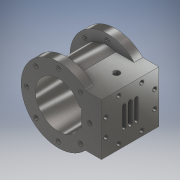
# Autodesk Inventor part: reverse gear cylinder
Saved by Autodesk Inventor 2017 (Build 210142000, 142)
## iProperties
Created: 2018-11-10
Part Number: reverse gear cylinder
Material: Generic
Document SubType Name: Modeling
Designer: User
Density: 1 g/cm^3
Appearance: Default
Author: User
Autodesk Inventor part; units mm, degrees
ref_plane "YZ Plane" through (0, 0, 0) normal (1, 0, 0) x (0, 1, 0)
sketch "Sketch2" plane through (0, 0, 0) normal (0, 1, 0) x (-1, 0, 0)
  arc A0 (-18.7617, -18) -> (-18.7617, 18) centre (0, 0) ccw
  arc A1 (-14.8324, -6) -> (-14.8324, 6) centre (0, 0) ccw
  line L0 (-16, 0) -> (-16, -6)
  line L1 (-16, 0) -> (-16, 6)
  line L2 (-16, 6) -> (-14.8324, 6) construction
  line L3 (-16, -6) -> (-14.8324, -6)
  circle A2 centre (22, 0) radius 1.5
  circle A3 centre (15.5563, 15.5563) radius 1.5
  circle A4 centre (0, 22) radius 1.5
  circle A5 centre (-15.5563, 15.5563) radius 1.5
  circle A6 centre (-22, 0) radius 1.5
  circle A7 centre (-15.5563, -15.5563) radius 1.5
  circle A8 centre (0, -22) radius 1.5
  circle A9 centre (15.5563, -15.5563) radius 1.5
  line L4 (-14.8324, 6) -> (-16, 6)
  line L5 (-30, 0) -> (-30, -18)
  line L6 (-30, -18) -> (-30, 18)
  line L7 (-30, 18) -> (-18.7617, 18)
  line L8 (-30, -18) -> (-18.7617, -18)
  arc A10 (-21.9489, 1.4991) -> (-22, 0) centre (0, 0) ccw
  line L9 (0, 0) -> (-16, 0)
  line L10 (-20.5, 0) -> (-22, 0)
  dimension "d10" = 360
  dimension "d2" = 52
  dimension "d3" = 32
  dimension "d4" = 6
  dimension "d5" = 6
  dimension "d6" = 3
  dimension "d7" = 30
  dimension "d8" = 18
  dimension "d9" = 36
  dimension "d36" = 22
  dimension "d37" = 0
  dimension "d38" = 18
  dimension "d39" = 0
  dimension "d40" = 16
  dimension "d41" = 38
  constraints: 22 end point, 11 centre point, 8 point on circle, 3 coincident, 3 equal length, 3 vertical, 2 horizontal, 2 perpendicular, 2 point on line, 2 tangent, 17 other
  measures "d2" diameter of A0
  measures "d3" diameter of A1
  measures "d4" distance of L0.start L0.end
  measures "d5" distance of L0.start L1.end
  measures "d6" diameter of A2
  measures "d7" distance of L9.start L5.start
  measures "d8" distance of L5.start L5.end
  measures "d9" distance of L5.end L6.end
  measures "d36" radius of A10
  measures "d37" distance between parallel lines of L10 L9
  measures "d38" distance between parallel lines of L9 L7
  measures "d39" distance from line of point (0, 0) L9
  measures "d40" distance from line of point (0, 0) L1
  measures "d41" distance from line of A2.centre L1
extrude "Extrusion1" add sketch "Sketch2" along normal blind 40
ref_plane "Work Plane1" through (0, 0, 0) normal (0, 1, 0) x (-1, 0, 0)
sketch "Sketch6" plane through (0, 0, 0) normal (0, 1, 0) x (-1, 0, 0)
  arc A0 (-6.0828, -18) -> (-6.0828, 18) centre (0, 0) ccw
  circle A1 centre (0, 0) radius 26
  arc A2 (-18.7617, -18) -> (-18.7617, 18) centre (0, 0) ccw
  line L0 (-18.7617, 18) -> (-6.0828, 18)
  line L1 (-18.7617, -18) -> (-6.0828, -18)
  dimension "d31" = 38
  dimension "d32" = 52
  dimension "d73" = 26
  dimension "d74" = 36
  dimension "d75" = 18
  dimension "d76" = 18
  dimension "d77" = 0
  constraints: 4 end point, 4 point on circle, 3 centre point, 2 coincident, 1 concentric, 1 horizontal, 1 parallel
  measures "d31" diameter of A0
  measures "d32" diameter of A1
  measures "d73" radius of A2
  measures "d74" distance between parallel lines of L1 L0
  measures "d75" distance from line of point (0, 0) L0
  measures "d76" distance from line of point (0, 0) L0
  measures "d77" distance of point (0, 0) A0.centre
sketch "Sketch4" plane through (30, 0, 18) normal (1, 0, 0) x (0, 0, -1)
  circle A0 centre (12, 3) radius 1.5
  circle A1 centre (3.5, 12) radius 1.5
  line L0 (0, 3) -> (0, 37) construction
  line L1 (0, 20) -> (36, 20) construction
  circle A2 centre (3.5, 28) radius 1.5
  circle A3 centre (12, 37) radius 1.5
  line L2 (16.5, 40) -> (19.5, 40) construction
  line L3 (18, 40) -> (18, 0) construction
  line L4 (19.5, 0) -> (16.5, 0) construction
  circle A4 centre (24, 37) radius 1.5
  circle A5 centre (32.5, 28) radius 1.5
  circle A6 centre (32.5, 12) radius 1.5
  circle A7 centre (24, 3) radius 1.5
  line L5 (-1, 37) -> (-1, 3)
  line L6 (37, 37) -> (37, 3)
  arc A8 (11.25, 21.5) -> (11.25, 18.5) centre (11.25, 20) ccw
  arc A9 (24.75, 18.5) -> (24.75, 21.5) centre (24.75, 20) ccw
  line L7 (24.75, 21.5) -> (24.75, 23)
  arc A10 (24.75, 23) -> (24.75, 25.5) centre (24.75, 24.25) ccw
  arc A11 (11.25, 25.5) -> (11.25, 23) centre (11.25, 24.25) ccw
  line L8 (24.75, 14.5) -> (11.25, 14.5)
  line L9 (24.75, 17) -> (11.25, 17)
  arc A12 (11.25, 17) -> (11.25, 14.5) centre (11.25, 15.75) ccw
  arc A13 (24.75, 14.5) -> (24.75, 17) centre (24.75, 15.75) ccw
  line L10 (11.25, 21.5) -> (24.75, 21.5)
  line L11 (24.75, 18.5) -> (11.25, 18.5)
  line L12 (11.25, 25.5) -> (24.75, 25.5)
  line L13 (11.25, 23) -> (24.75, 23)
  point P0 (18, 0)
  point P1 (0, 40)
  point P2 (36, 3)
  point P3 (18, 0)
  dimension "d18" = 3
  dimension "d21" = 3
  dimension "d22" = 3
  dimension "d23" = 1.5
  dimension "d24" = 2.5
  dimension "d25" = 2.5
  dimension "d26" = 2.5
  dimension "d42" = 12.25
  dimension "d43" = 19
  dimension "d44" = 37
  dimension "d45" = 38
  dimension "d46" = 25.5
  dimension "d47" = 20
  dimension "d48" = 17
  dimension "d49" = 40
  dimension "d50" = 19
  dimension "d51" = 0
  dimension "d52" = 37
  dimension "d53" = 3
  dimension "d54" = 1
  dimension "d55" = 1
  dimension "d56" = 3
  dimension "d57" = 4.5
  dimension "d58" = 28
  dimension "d59" = 12.25
  dimension "d60" = 13
  dimension "d61" = 37
  dimension "d62" = 17.5
  dimension "d63" = 17.5
  dimension "d64" = 19
  dimension "d65" = 0
  dimension "d66" = 25.75
  dimension "d67" = 25.75
  dimension "d68" = 37
  dimension "d69" = 40
  dimension "d70" = 37
  dimension "d71" = 37
  dimension "d72" = 3
  constraints: 28 end point, 14 centre point, 12 point on circle, 12 tangent, 9 parallel, 6 symmetric about line, 3 midpoint, 2 equal radius, 2 horizontal, 1 vertical, 6 other
  measures "d18" diameter of A0
  measures "d21" diameter of A8
  measures "d22" diameter of A9
  measures "d23" distance of L7.start L7.end
  measures "d24" distance of L12.end L7.end
  measures "d25" diameter of A10
  measures "d26" diameter of A11
  measures "d42" distance between parallel lines of L6 L7
  measures "d43" distance between parallel lines of L3 L6
  measures "d44" distance between parallel lines of L0 L6
  measures "d45" distance between parallel lines of L5 L6
  measures "d46" distance between parallel lines of L4 L12
  measures "d47" distance between parallel lines of L4 L1
  measures "d48" distance between parallel lines of L4 L9
  measures "d49" distance between parallel lines of L4 L2
  measures "d50" distance from line of point (18, 0) L6
  measures "d51" distance from line of point (18, 0) L4
  measures "d52" distance from line of L6.start L4
  measures "d53" distance from line of L6.end L4
  measures "d54" distance from line of L1.end L6
  measures "d55" distance from line of point (36, 3) L6
  measures "d56" distance from line of point (36, 3) L4
  measures "d57" distance from line of A5.centre L6
  measures "d58" distance from line of A5.centre L4
  measures "d59" distance from line of L9.start L6
  measures "d60" distance from line of A4.centre L6
  measures "d61" distance from line of A4.centre L4
  measures "d62" distance from line of L2.end L6
  measures "d63" distance from line of L4.start L6
  measures "d64" distance from line of point (18, 0) L6
  measures "d65" distance from line of point (18, 0) L4
  measures "d66" distance from line of L10.start L6
  measures "d67" distance from line of L9.end L6
  measures "d68" distance from line of point (0, 40) L6
  measures "d69" distance from line of point (0, 40) L4
  measures "d70" distance from line of L0.end L4
  measures "d71" distance from line of L5.start L4
  measures "d72" distance from line of L5.end L4
extrude "Extrusion5" cut sketch "Sketch4" against normal blind 11
extrude "Extrusion6" cut sketch "Sketch6" along normal blind 34 contours A0 L0 A1 L1 picked at (-12.9468, 19.3038)
ref_plane "Work Plane2" through (0, 20, 0) normal (0, 1, 0) x (-1, 0, 0)
mirror "Mirror1" about plane through (0, 20, 0) normal (0, 1, 0)
sketch "Sketch9" plane through (18.7617, 40, 18) normal (0, 0, 1) x (1, 0, 0)
  line L0 (-12.6789, -34) -> (0, -34) projected
  line L1 (0, -34) -> (0, -40) projected
  line L2 (11.2383, -40) -> (0, -40) projected
  line L3 (11.2383, -40) -> (11.2383, 0) projected
  line L4 (0, 0) -> (11.2383, 0) projected
  line L5 (0, -6) -> (0, 0) projected
  line L6 (0, -6) -> (-12.6789, -6) projected
  line L7 (-12.6789, -34) -> (-12.6789, -6) projected
  line L8 (11.2383, -18.5) -> (0.2383, -18.5) projected
  circle A0 centre (0.2383, -18.5) radius 2.25
  point P0 (-18.7617, -40)
  dimension "d81" = 4.5
  constraints: 1 centre point, 1 coincident
  measures "d81" diameter of A0
extrude "Extrusion8" cut sketch "Sketch9" against normal blind 10 contours A0
body "Solid1"
